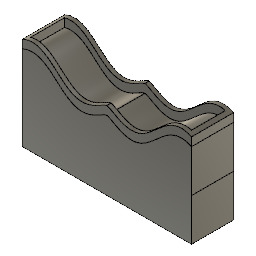
Hill V1 v1 (Autodesk Fusion 360 design; units mm, degrees)
Autodesk Fusion 360 part; units mm, degrees
sketch "Sketch1" plane through (0, 0, 0) normal (0, 1, 0) x (1, 0, 0)
  line L0 (-100, 0) -> (100, 0)
  line L1 (100, 0) -> (100, -50)
  line L2 (-100, 0) -> (-100, -50)
  line L3 (-100, -50) -> (-100, -100)
  spline S0 degree 5 poles (-100, -100) (-98.8521, -100.5535) (-96.5633, -101.53) (-93.1507, -102.6036) (-88.642, -103.2494) (-83.0742, -102.7477) (-77.5698, -100.9702) (-72.1177, -98.0117) (-66.6988, -94.0524) (-61.2812, -89.3993) (-55.8236, -84.4793) (-50.2867, -79.7684) (-44.6439, -75.7365) (-38.8917, -72.7869) (-33.0614, -71.1949) (-27.2293, -71.0491) (-21.5329, -72.1705) (-16.1509, -74.1814) (-11.2758, -76.6036) (-7.0886, -78.949) (-3.7347, -80.801) (-1.7785, -81.7011) (-0.7267, -82.0208) (-0.2095, -82.0762) (0.0031, -82.0645) knots 0 0 0 0 0 0 0.05 0.1 0.15 0.2 0.25 0.3 0.35 0.4 0.45 0.5 0.55 0.6 0.65 0.7 0.75 0.8 0.85 0.9 0.95 1 1 1 1 1 1
  line L4 (20.0031, -142.0645) -> (20.0031, -153.756)
  spline S1 degree 5 poles (100.0061, -100) (98.8583, -100.5535) (96.5694, -101.53) (93.1568, -102.6036) (88.6481, -103.2494) (83.0803, -102.7477) (77.5759, -100.9702) (72.1238, -98.0117) (66.7049, -94.0524) (61.2873, -89.3993) (55.8297, -84.4793) (50.2928, -79.7684) (44.65, -75.7365) (38.8978, -72.7869) (33.0675, -71.1949) (27.2354, -71.0491) (21.539, -72.1705) (16.157, -74.1814) (11.282, -76.6036) (7.0948, -78.949) (3.7408, -80.801) (1.7846, -81.7011) (0.7328, -82.0208) (0.2157, -82.0762) (0.0031, -82.0645) knots 0 0 0 0 0 0 0.05 0.1 0.15 0.2 0.25 0.3 0.35 0.4 0.45 0.5 0.55 0.6 0.65 0.7 0.75 0.8 0.85 0.9 0.95 1 1 1 1 1 1
  line L5 (110.8987, -94.7479) -> (89.1136, -105.2521)
  line L6 (4.8088, -82.3291) -> (-4.8026, -81.7998)
  line L7 (100, -50) -> (100.0061, -100)
  spline S2 degree 5 poles (-100, -130) (-98.8521, -130.5535) (-96.5633, -131.53) (-93.1507, -132.6036) (-88.642, -133.2494) (-83.0742, -132.7477) (-77.5698, -130.9702) (-72.1177, -128.0117) (-66.6988, -124.0524) (-61.2812, -119.3993) (-55.8236, -114.4793) (-50.2867, -109.7684) (-44.6439, -105.7365) (-38.8917, -102.7869) (-33.0614, -101.1949) (-27.2293, -101.0491) (-21.5329, -102.1705) (-16.1509, -104.1814) (-11.2758, -106.6036) (-7.0886, -108.949) (-3.7347, -110.801) (-1.7785, -111.7011) (-0.7267, -112.0208) (-0.2095, -112.0762) (0.0031, -112.0645) knots 0 0 0 0 0 0 0.05 0.1 0.15 0.2 0.25 0.3 0.35 0.4 0.45 0.5 0.55 0.6 0.65 0.7 0.75 0.8 0.85 0.9 0.95 1 1 1 1 1 1
  spline S3 degree 5 poles (100.0061, -130) (98.8583, -130.5535) (96.5694, -131.53) (93.1568, -132.6036) (88.6481, -133.2494) (83.0803, -132.7477) (77.5759, -130.9702) (72.1238, -128.0117) (66.7049, -124.0524) (61.2873, -119.3993) (55.8297, -114.4793) (50.2928, -109.7684) (44.65, -105.7365) (38.8978, -102.7869) (33.0675, -101.1949) (27.2354, -101.0491) (21.539, -102.1705) (16.157, -104.1814) (11.282, -106.6036) (7.0948, -108.949) (3.7408, -110.801) (1.7846, -111.7011) (0.7328, -112.0208) (0.2157, -112.0762) (0.0031, -112.0645) knots 0 0 0 0 0 0 0.05 0.1 0.15 0.2 0.25 0.3 0.35 0.4 0.45 0.5 0.55 0.6 0.65 0.7 0.75 0.8 0.85 0.9 0.95 1 1 1 1 1 1
  line L8 (110.8987, -124.7479) -> (89.1136, -135.2521)
  line L9 (4.8088, -112.3291) -> (-4.8026, -111.7998)
  spline S4 degree 5 poles (-100, -140) (-98.8521, -140.5535) (-96.5633, -141.53) (-93.1507, -142.6036) (-88.642, -143.2494) (-83.0742, -142.7477) (-77.5698, -140.9702) (-72.1177, -138.0117) (-66.6988, -134.0524) (-61.2812, -129.3993) (-55.8236, -124.4793) (-50.2867, -119.7684) (-44.6439, -115.7365) (-38.8917, -112.7869) (-33.0614, -111.1949) (-27.2293, -111.0491) (-21.5329, -112.1705) (-16.1509, -114.1814) (-11.2758, -116.6036) (-7.0886, -118.949) (-3.7347, -120.801) (-1.7785, -121.7011) (-0.7267, -122.0208) (-0.2095, -122.0762) (0.0031, -122.0645) knots 0 0 0 0 0 0 0.05 0.1 0.15 0.2 0.25 0.3 0.35 0.4 0.45 0.5 0.55 0.6 0.65 0.7 0.75 0.8 0.85 0.9 0.95 1 1 1 1 1 1
  spline S5 degree 5 poles (100.0061, -140) (98.8583, -140.5535) (96.5694, -141.53) (93.1568, -142.6036) (88.6481, -143.2494) (83.0803, -142.7477) (77.5759, -140.9702) (72.1238, -138.0117) (66.7049, -134.0524) (61.2873, -129.3993) (55.8297, -124.4793) (50.2928, -119.7684) (44.65, -115.7365) (38.8978, -112.7869) (33.0675, -111.1949) (27.2354, -111.0491) (21.539, -112.1705) (16.157, -114.1814) (11.282, -116.6036) (7.0948, -118.949) (3.7408, -120.801) (1.7846, -121.7011) (0.7328, -122.0208) (0.2157, -122.0762) (0.0031, -122.0645) knots 0 0 0 0 0 0 0.05 0.1 0.15 0.2 0.25 0.3 0.35 0.4 0.45 0.5 0.55 0.6 0.65 0.7 0.75 0.8 0.85 0.9 0.95 1 1 1 1 1 1
  line L10 (110.8987, -134.7479) -> (89.1136, -145.2521)
  line L11 (4.8088, -122.3291) -> (-4.8026, -121.7998)
  line L12 (-100, -140) -> (-100, -130)
  line L13 (100.0061, -140) -> (100.0061, -130)
  point P0 (-68.9885, -95.6207)
  point P1 (-31.9509, -71.4132)
  point P2 (-5.8068, -79.6437)
  point P3 (68.9946, -95.6207)
  point P4 (31.957, -71.4132)
  point P5 (5.8129, -79.6437)
  point P6 (68.9946, -125.6207)
  point P7 (31.957, -101.4132)
  point P8 (5.8129, -109.6437)
  point P9 (-31.9509, -101.4132)
  point P10 (-5.8068, -109.6437)
  point P11 (-68.9885, -125.6207)
  point P12 (-68.9885, -135.6207)
  point P13 (31.957, -111.4132)
  point P14 (5.8129, -119.6437)
  point P15 (-5.8068, -119.6437)
  point P16 (68.9946, -135.6207)
  point P17 (-31.9509, -111.4132)
  constraint horizontal L0
  constraint perpendicular L0 L1
  constraint perpendicular L0 L2
  constraint parallel L2 L3
  constraint vertical L4
  constraint vertical L12
  constraint parallel L12 L13
extrude "Extrude1" add sketch "Sketch1" along normal blind 50 contours L0 L1 L2 L3 S0 S1 L6 L7 | S0 L6 | S2 S3 S4 S5 L11 L12 L13 | S4 L11 makes body 1 at (-63.5321, 15.2778, 121.2812) makes body 2 at (-7.9492, 0, 23.9512)
move_body "Move1" bodies 1 to x (1, 0, 0) y (0, 1, 0) z (0, 0, 1) at (0, 0, 30)
ref_plane "WorkPlane1" through (0, 0, 120) normal (0, 0, 1) x (1, 0, 0)
sketch "Sketch3" plane through (0, 0, 120) normal (0, 0, 1) x (1, 0, 0)
  line L0 (100, 0) -> (100, 5)
  line L1 (100, 5) -> (95, 5)
  line L2 (95, 5) -> (95, 45)
  line L3 (95, 5) -> (-95, 5)
  line L4 (95, 45) -> (-95, 45)
  line L5 (-95, 45) -> (-95, 5)
  dimension "d4" = 5
  dimension "d5" = 5
  dimension "d6" = 40
  dimension "d7" = 190
  constraint vertical L0
  constraint perpendicular L0 L1
  constraint perpendicular L1 L2
  constraint perpendicular L2 L3
  constraint perpendicular L2 L4
  constraint perpendicular L3 L5
  measures "d4" distance of L0.start L0.end
  measures "d5" distance of L0.end L1.end
  measures "d6" distance of L1.end L2.end
  measures "d7" distance of L1.end L3.end
extrude "Extrude2" cut sketch "Sketch3" along normal blind 70 bodies 1
move_body "Move2" bodies 1 to x (1, 0, 0) y (0, 1, 0) z (0, 0, 1) at (0, 0, -60)
